Autodesk Inventor part; units mm, degrees
(part 2 of 2)
sketch "Sketch2" plane through (0, 0, 2.286) normal (0, 0, 1) x (1, 0, 0)
  line L0 (711.2, 0) -> (711.2, -863.6) projected
  line L1 (0, 0) -> (711.2, 0) projected
  line L2 (0, -863.6) -> (0, 0) projected
  point P0 (12.7, -12.7)
  point P1 (114.3, -12.7)
  point P2 (596.9, -12.7)
  point P3 (698.5, -12.7)
  point P4 (12.7, -38.1)
  point P5 (114.3, -38.1)
  point P6 (596.9, -38.1)
  point P7 (698.5, -38.1)
  point P8 (12.7, -63.5)
  point P9 (114.3, -63.5)
  point P10 (596.9, -63.5)
  point P11 (698.5, -63.5)
  point P12 (12.7, -88.9)
  point P13 (114.3, -88.9)
  point P14 (596.9, -88.9)
  point P15 (698.5, -88.9)
  point P16 (12.7, -114.3)
  point P17 (114.3, -114.3)
  point P18 (596.9, -114.3)
  point P19 (698.5, -114.3)
  point P20 (12.7, -139.7)
  point P21 (114.3, -139.7)
  point P22 (596.9, -139.7)
  point P23 (698.5, -139.7)
  point P24 (12.7, -165.1)
  point P25 (114.3, -165.1)
  point P26 (596.9, -165.1)
  point P27 (698.5, -165.1)
  point P28 (12.7, -190.5)
  point P29 (114.3, -190.5)
  point P30 (596.9, -190.5)
  point P31 (698.5, -190.5)
  point P32 (12.7, -215.9)
  point P33 (114.3, -215.9)
  point P34 (596.9, -215.9)
  point P35 (698.5, -215.9)
  point P36 (12.7, -241.3)
  point P37 (114.3, -241.3)
  point P38 (596.9, -241.3)
  point P39 (698.5, -241.3)
  point P40 (12.7, -266.7)
  point P41 (114.3, -266.7)
  point P42 (596.9, -266.7)
  point P43 (698.5, -266.7)
  point P44 (12.7, -292.1)
  point P45 (114.3, -292.1)
  point P46 (596.9, -292.1)
  point P47 (698.5, -292.1)
  point P48 (12.7, -317.5)
  point P49 (114.3, -317.5)
  point P50 (596.9, -317.5)
  point P51 (698.5, -317.5)
  point P52 (12.7, -342.9)
  point P53 (114.3, -342.9)
  point P54 (596.9, -342.9)
  point P55 (698.5, -342.9)
  point P56 (12.7, -368.3)
  point P57 (114.3, -368.3)
  point P58 (596.9, -368.3)
  point P59 (698.5, -368.3)
  point P60 (12.7, -393.7)
  point P61 (114.3, -393.7)
  point P62 (596.9, -393.7)
  point P63 (698.5, -393.7)
  point P64 (12.7, -419.1)
  point P65 (114.3, -419.1)
  point P66 (596.9, -419.1)
  point P67 (698.5, -419.1)
  point P68 (12.7, -444.5)
  point P69 (114.3, -444.5)
  point P70 (596.9, -444.5)
  point P71 (698.5, -444.5)
  point P72 (12.7, -469.9)
  point P73 (114.3, -469.9)
  point P74 (596.9, -469.9)
  point P75 (698.5, -469.9)
  point P76 (12.7, -495.3)
  point P77 (114.3, -495.3)
  point P78 (596.9, -495.3)
  point P79 (698.5, -495.3)
  point P80 (12.7, -520.7)
  point P81 (114.3, -520.7)
  point P82 (596.9, -520.7)
  point P83 (698.5, -520.7)
  point P84 (12.7, -546.1)
  point P85 (114.3, -546.1)
  point P86 (596.9, -546.1)
  point P87 (698.5, -546.1)
  point P88 (12.7, -571.5)
  point P89 (114.3, -571.5)
  point P90 (596.9, -571.5)
  point P91 (698.5, -571.5)
  point P92 (12.7, -596.9)
  point P93 (114.3, -596.9)
  point P94 (596.9, -596.9)
  point P95 (698.5, -596.9)
  point P96 (12.7, -622.3)
  point P97 (114.3, -622.3)
  point P98 (596.9, -622.3)
  point P99 (698.5, -622.3)
  point P100 (12.7, -647.7)
  point P101 (114.3, -647.7)
  point P102 (596.9, -647.7)
  point P103 (698.5, -647.7)
  point P104 (12.7, -673.1)
  point P105 (114.3, -673.1)
  point P106 (596.9, -673.1)
  point P107 (698.5, -673.1)
  point P108 (12.7, -698.5)
  point P109 (114.3, -698.5)
  point P110 (596.9, -698.5)
  point P111 (698.5, -698.5)
  point P112 (12.7, -723.9)
  point P113 (114.3, -723.9)
  point P114 (596.9, -723.9)
  point P115 (698.5, -723.9)
  point P116 (12.7, -749.3)
  point P117 (114.3, -749.3)
  point P118 (596.9, -749.3)
  point P119 (698.5, -749.3)
  point P120 (12.7, -774.7)
  point P121 (114.3, -774.7)
  point P122 (596.9, -774.7)
  point P123 (698.5, -774.7)
  point P124 (12.7, -800.1)
  point P125 (114.3, -800.1)
  point P126 (596.9, -800.1)
  point P127 (698.5, -800.1)
  point P128 (12.7, -825.5)
  point P129 (114.3, -825.5)
  point P130 (596.9, -825.5)
  point P131 (698.5, -825.5)
  point P132 (12.7, -850.9)
  point P133 (114.3, -850.9)
  point P134 (596.9, -850.9)
  point P135 (698.5, -850.9)
  dimension "d37" = 12.7
  dimension "d38" = 114.3
  dimension "d39" = 114.3
  dimension "d40" = 12.7
  dimension "d41" = 12.7
  dimension "d44" = 25.4
  constraints: 3 horizontal alignment, 1 vertical, 132 other
  measures "d37" distance from line of L2 point (12.7, -12.7)
  measures "d38" distance from line of L2 point (114.3, -12.7)
  measures "d39" distance from line of L0 point (596.9, -12.7)
  measures "d40" distance from line of L0 point (698.5, -12.7)
  measures "d41" distance from line of L1 point (698.5, -12.7)
  measures "d44" distance of point (698.5, -12.7) point (698.5, -38.1)
hole "Hole1" at (12.7, -12.7, 2.286) at (114.3, -12.7, 2.286) at (596.9, -12.7, 2.286) at (698.5, -12.7, 2.286) at (698.5, -38.1, 2.286) at (596.9, -38.1, 2.286) at (114.3, -38.1, 2.286) at (12.7, -38.1, 2.286) at (698.5, -63.5, 2.286) at (596.9, -63.5, 2.286) at (114.3, -63.5, 2.286) at (12.7, -63.5, 2.286) at (698.5, -88.9, 2.286) at (596.9, -88.9, 2.286) at (114.3, -88.9, 2.286) at (12.7, -88.9, 2.286) at (698.5, -114.3, 2.286) at (596.9, -114.3, 2.286) at (114.3, -114.3, 2.286) at (12.7, -114.3, 2.286) at (698.5, -139.7, 2.286) at (596.9, -139.7, 2.286) at (114.3, -139.7, 2.286) at (12.7, -139.7, 2.286) at (698.5, -165.1, 2.286) at (596.9, -165.1, 2.286) at (114.3, -165.1, 2.286) at (12.7, -165.1, 2.286) at (698.5, -190.5, 2.286) at (596.9, -190.5, 2.286) at (114.3, -190.5, 2.286) at (12.7, -190.5, 2.286) at (698.5, -215.9, 2.286) at (596.9, -215.9, 2.286) at (114.3, -215.9, 2.286) at (12.7, -215.9, 2.286) at (698.5, -241.3, 2.286) at (596.9, -241.3, 2.286) at (114.3, -241.3, 2.286) at (12.7, -241.3, 2.286) at (698.5, -266.7, 2.286) at (596.9, -266.7, 2.286) at (114.3, -266.7, 2.286) at (12.7, -266.7, 2.286) at (698.5, -292.1, 2.286) at (596.9, -292.1, 2.286) at (114.3, -292.1, 2.286) at (12.7, -292.1, 2.286) at (698.5, -317.5, 2.286) at (596.9, -317.5, 2.286) direction (0, 0, -1) diameter 6.7564 end through all and at (114.3, -317.5, 2.286) (12.7, -317.5, 2.286) (698.5, -342.9, 2.286) (596.9, -342.9, 2.286) (114.3, -342.9, 2.286) (12.7, -342.9, 2.286) (698.5, -368.3, 2.286) (596.9, -368.3, 2.286) (114.3, -368.3, 2.286) (12.7, -368.3, 2.286) (698.5, -393.7, 2.286) (596.9, -393.7, 2.286) (114.3, -393.7, 2.286) (12.7, -393.7, 2.286) (698.5, -419.1, 2.286) (596.9, -419.1, 2.286) (114.3, -419.1, 2.286) (12.7, -419.1, 2.286) (698.5, -444.5, 2.286) (596.9, -444.5, 2.286) (114.3, -444.5, 2.286) (12.7, -444.5, 2.286) (698.5, -469.9, 2.286) (596.9, -469.9, 2.286) (114.3, -469.9, 2.286) (12.7, -469.9, 2.286) (698.5, -495.3, 2.286) (596.9, -495.3, 2.286) (114.3, -495.3, 2.286) (12.7, -495.3, 2.286) (698.5, -520.7, 2.286) (596.9, -520.7, 2.286) (114.3, -520.7, 2.286) (12.7, -520.7, 2.286) (698.5, -546.1, 2.286) (596.9, -546.1, 2.286) (114.3, -546.1, 2.286) (12.7, -546.1, 2.286) (698.5, -571.5, 2.286) (596.9, -571.5, 2.286) (114.3, -571.5, 2.286) (12.7, -571.5, 2.286) (698.5, -596.9, 2.286) (596.9, -596.9, 2.286) (114.3, -596.9, 2.286) (12.7, -596.9, 2.286) (698.5, -622.3, 2.286) (596.9, -622.3, 2.286) (114.3, -622.3, 2.286) (12.7, -622.3, 2.286) (698.5, -647.7, 2.286) (596.9, -647.7, 2.286) (114.3, -647.7, 2.286) (12.7, -647.7, 2.286) (698.5, -673.1, 2.286) (596.9, -673.1, 2.286) (114.3, -673.1, 2.286) (12.7, -673.1, 2.286) (698.5, -698.5, 2.286) (596.9, -698.5, 2.286) (114.3, -698.5, 2.286) (12.7, -698.5, 2.286) (698.5, -723.9, 2.286) (596.9, -723.9, 2.286) (114.3, -723.9, 2.286) (12.7, -723.9, 2.286) (698.5, -749.3, 2.286) (596.9, -749.3, 2.286) (114.3, -749.3, 2.286) (12.7, -749.3, 2.286) (698.5, -774.7, 2.286) (596.9, -774.7, 2.286) (114.3, -774.7, 2.286) (12.7, -774.7, 2.286) (698.5, -800.1, 2.286) (596.9, -800.1, 2.286) (114.3, -800.1, 2.286) (12.7, -800.1, 2.286) (698.5, -825.5, 2.286) (596.9, -825.5, 2.286) (114.3, -825.5, 2.286) (12.7, -825.5, 2.286) (698.5, -850.9, 2.286) (596.9, -850.9, 2.286) (114.3, -850.9, 2.286) (12.7, -850.9, 2.286)
sketch "Sketch3" plane through (0, 0, 2.286) normal (0, 0, 1) x (1, 0, 0)
  line L0 (0, 0) -> (711.2, 0) projected
  line L1 (0, -863.6) -> (0, 0) projected
  line L2 (34.925, -38.1) -> (92.075, -38.1)
  line L3 (95.25, -41.275) -> (95.25, -161.925)
  line L4 (92.075, -165.1) -> (34.925, -165.1)
  line L5 (31.75, -161.925) -> (31.75, -41.275)
  arc A0 (34.925, -38.1) -> (31.75, -41.275) centre (34.925, -41.275) ccw
  arc A1 (31.75, -161.925) -> (34.925, -165.1) centre (34.925, -161.925) ccw
  arc A2 (92.075, -165.1) -> (95.25, -161.925) centre (92.075, -161.925) ccw
  arc A3 (95.25, -41.275) -> (92.075, -38.1) centre (92.075, -41.275) ccw
  line L6 (34.925, -203.2) -> (92.075, -203.2)
  line L7 (95.25, -206.375) -> (95.25, -327.025)
  line L8 (92.075, -330.2) -> (34.925, -330.2)
  line L9 (31.75, -327.025) -> (31.75, -206.375)
  arc A4 (34.925, -203.2) -> (31.75, -206.375) centre (34.925, -206.375) ccw
  arc A5 (31.75, -327.025) -> (34.925, -330.2) centre (34.925, -327.025) ccw
  arc A6 (92.075, -330.2) -> (95.25, -327.025) centre (92.075, -327.025) ccw
  arc A7 (95.25, -206.375) -> (92.075, -203.2) centre (92.075, -206.375) ccw
  line L10 (34.925, -368.3) -> (92.075, -368.3)
  line L11 (95.25, -371.475) -> (95.25, -492.125)
  line L12 (92.075, -495.3) -> (34.925, -495.3)
  line L13 (31.75, -492.125) -> (31.75, -371.475)
  arc A8 (34.925, -368.3) -> (31.75, -371.475) centre (34.925, -371.475) ccw
  arc A9 (31.75, -492.125) -> (34.925, -495.3) centre (34.925, -492.125) ccw
  arc A10 (92.075, -495.3) -> (95.25, -492.125) centre (92.075, -492.125) ccw
  arc A11 (95.25, -371.475) -> (92.075, -368.3) centre (92.075, -371.475) ccw
  line L14 (34.925, -533.4) -> (92.075, -533.4)
  line L15 (95.25, -536.575) -> (95.25, -657.225)
  line L16 (92.075, -660.4) -> (34.925, -660.4)
  line L17 (31.75, -657.225) -> (31.75, -536.575)
  arc A12 (34.925, -533.4) -> (31.75, -536.575) centre (34.925, -536.575) ccw
  arc A13 (31.75, -657.225) -> (34.925, -660.4) centre (34.925, -657.225) ccw
  arc A14 (92.075, -660.4) -> (95.25, -657.225) centre (92.075, -657.225) ccw
  arc A15 (95.25, -536.575) -> (92.075, -533.4) centre (92.075, -536.575) ccw
  line L18 (34.925, -698.5) -> (92.075, -698.5)
  line L19 (95.25, -701.675) -> (95.25, -822.325)
  line L20 (92.075, -825.5) -> (34.925, -825.5)
  line L21 (31.75, -822.325) -> (31.75, -701.675)
  arc A16 (34.925, -698.5) -> (31.75, -701.675) centre (34.925, -701.675) ccw
  arc A17 (31.75, -822.325) -> (34.925, -825.5) centre (34.925, -822.325) ccw
  arc A18 (92.075, -825.5) -> (95.25, -822.325) centre (92.075, -822.325) ccw
  arc A19 (95.25, -701.675) -> (92.075, -698.5) centre (92.075, -701.675) ccw
  line L22 (619.125, -38.1) -> (676.275, -38.1)
  line L23 (679.45, -41.275) -> (679.45, -161.925)
  line L24 (676.275, -165.1) -> (619.125, -165.1)
  line L25 (615.95, -161.925) -> (615.95, -41.275)
  arc A20 (619.125, -38.1) -> (615.95, -41.275) centre (619.125, -41.275) ccw
  arc A21 (615.95, -161.925) -> (619.125, -165.1) centre (619.125, -161.925) ccw
  arc A22 (676.275, -165.1) -> (679.45, -161.925) centre (676.275, -161.925) ccw
  arc A23 (679.45, -41.275) -> (676.275, -38.1) centre (676.275, -41.275) ccw
  line L26 (619.125, -203.2) -> (676.275, -203.2)
  line L27 (679.45, -206.375) -> (679.45, -327.025)
  line L28 (676.275, -330.2) -> (619.125, -330.2)
  line L29 (615.95, -327.025) -> (615.95, -206.375)
  arc A24 (619.125, -203.2) -> (615.95, -206.375) centre (619.125, -206.375) ccw
  arc A25 (615.95, -327.025) -> (619.125, -330.2) centre (619.125, -327.025) ccw
  arc A26 (676.275, -330.2) -> (679.45, -327.025) centre (676.275, -327.025) ccw
  arc A27 (679.45, -206.375) -> (676.275, -203.2) centre (676.275, -206.375) ccw
  line L30 (619.125, -368.3) -> (676.275, -368.3)
  line L31 (679.45, -371.475) -> (679.45, -492.125)
  line L32 (676.275, -495.3) -> (619.125, -495.3)
  line L33 (615.95, -492.125) -> (615.95, -371.475)
  arc A28 (619.125, -368.3) -> (615.95, -371.475) centre (619.125, -371.475) ccw
  arc A29 (615.95, -492.125) -> (619.125, -495.3) centre (619.125, -492.125) ccw
  arc A30 (676.275, -495.3) -> (679.45, -492.125) centre (676.275, -492.125) ccw
  arc A31 (679.45, -371.475) -> (676.275, -368.3) centre (676.275, -371.475) ccw
  line L34 (619.125, -533.4) -> (676.275, -533.4)
  line L35 (679.45, -536.575) -> (679.45, -657.225)
  line L36 (676.275, -660.4) -> (619.125, -660.4)
  line L37 (615.95, -657.225) -> (615.95, -536.575)
  arc A32 (619.125, -533.4) -> (615.95, -536.575) centre (619.125, -536.575) ccw
  arc A33 (615.95, -657.225) -> (619.125, -660.4) centre (619.125, -657.225) ccw
  arc A34 (676.275, -660.4) -> (679.45, -657.225) centre (676.275, -657.225) ccw
  arc A35 (679.45, -536.575) -> (676.275, -533.4) centre (676.275, -536.575) ccw
  line L38 (619.125, -698.5) -> (676.275, -698.5)
  line L39 (679.45, -701.675) -> (679.45, -822.325)
  line L40 (676.275, -825.5) -> (619.125, -825.5)
  line L41 (615.95, -822.325) -> (615.95, -701.675)
  arc A36 (619.125, -698.5) -> (615.95, -701.675) centre (619.125, -701.675) ccw
  arc A37 (615.95, -822.325) -> (619.125, -825.5) centre (619.125, -822.325) ccw
  arc A38 (676.275, -825.5) -> (679.45, -822.325) centre (676.275, -822.325) ccw
  arc A39 (679.45, -701.675) -> (676.275, -698.5) centre (676.275, -701.675) ccw
  point P0 (31.75, -38.1)
  point P1 (31.75, -165.1)
  point P2 (31.75, -203.2)
  point P3 (31.75, -330.2)
  point P4 (31.75, -368.3)
  point P5 (31.75, -495.3)
  point P6 (31.75, -533.4)
  point P7 (31.75, -660.4)
  point P8 (31.75, -698.5)
  point P9 (31.75, -825.5)
  point P10 (615.95, -38.1)
  point P11 (615.95, -165.1)
  point P12 (615.95, -203.2)
  point P13 (615.95, -330.2)
  point P14 (615.95, -368.3)
  point P15 (615.95, -495.3)
  point P16 (615.95, -533.4)
  point P17 (615.95, -660.4)
  point P18 (615.95, -698.5)
  point P19 (615.95, -825.5)
  dimension "d56" = 31.75
  dimension "d57" = 38.1
  dimension "d58" = 95.25
  dimension "d59" = 127
  dimension "d60" = 3.175
  dimension "d63" = 165.1
  dimension "d66" = 584.2
  constraints: 80 end point, 80 point on circle, 40 centre point, 40 point on line, 8 tangent, 3 equal radius, 2 horizontal, 2 parallel, 1 perpendicular, 1 vertical, 198 other
  measures "d56" distance between parallel lines of L1 L5
  measures "d57" distance between parallel lines of L0 L2
  measures "d58" distance between parallel lines of L1 L3
  measures "d59" distance of point (31.75, -165.1) point (31.75, -38.1)
  measures "d60" radius of A0
  measures "d63" distance of point (31.75, -165.1) point (31.75, -330.2)
  measures "d66" distance of point (31.75, -165.1) point (615.95, -165.1)
extrude "Cut1" cut sketch "Sketch3" against normal blind 3.048
sketch "Sketch4" plane through (0, 0, 2.286) normal (0, 0, 1) x (1, 0, 0)
  line L0 (190.5, -234.8865) -> (142.9908, -163.6227) projected
  arc A0 (145.6325, -158.6865) -> (142.9908, -163.6227) centre (145.6325, -161.8615) ccw projected
  line L1 (145.6325, -158.6865) -> (187.325, -158.6865) projected
  arc A1 (190.5, -161.8615) -> (187.325, -158.6865) centre (187.325, -161.8615) ccw projected
  line L2 (190.5, -161.8615) -> (190.5, -234.8865) projected
  arc A2 (187.325, -145.9865) -> (190.5, -142.8115) centre (187.325, -142.8115) ccw projected
  line L3 (187.325, -145.9865) -> (145.6325, -145.9865) projected
  arc A3 (142.9908, -141.0503) -> (145.6325, -145.9865) centre (145.6325, -142.8115) ccw projected
  line L4 (142.9908, -141.0503) -> (190.5, -69.7865) projected
  line L5 (190.5, -69.7865) -> (190.5, -142.8115) projected
  arc A4 (571.5, -161.8615) -> (568.325, -158.6865) centre (568.325, -161.8615) ccw projected
  line L6 (571.5, -161.8615) -> (571.5, -224.4002) projected
  arc A5 (565.6832, -226.1614) -> (571.5, -224.4002) centre (568.325, -224.4002) ccw projected
  line L7 (565.6832, -226.1614) -> (523.9908, -163.6227) projected
  arc A6 (526.6325, -158.6865) -> (523.9908, -163.6227) centre (526.6325, -161.8615) ccw projected
  line L8 (526.6325, -158.6865) -> (568.325, -158.6865) projected
  arc A7 (142.875, -46.9011) -> (139.7, -50.0761) centre (142.875, -50.0761) ccw projected
  line L9 (142.875, -46.9011) -> (184.5675, -46.9011) projected
  arc A8 (187.2092, -51.8373) -> (184.5675, -46.9011) centre (184.5675, -50.0761) ccw projected
  line L10 (187.2092, -51.8373) -> (145.5168, -114.376) projected
  arc A9 (139.7, -112.6148) -> (145.5168, -114.376) centre (142.875, -112.6148) ccw projected
  line L11 (139.7, -112.6148) -> (139.7, -50.0761) projected
  arc A10 (523.875, -46.9011) -> (520.7, -50.0761) centre (523.875, -50.0761) ccw projected
  line L12 (523.875, -46.9011) -> (565.5675, -46.9011) projected
  arc A11 (568.2092, -51.8373) -> (565.5675, -46.9011) centre (565.5675, -50.0761) ccw projected
  line L13 (568.2092, -51.8373) -> (526.5168, -114.376) projected
  arc A12 (520.7, -112.6148) -> (526.5168, -114.376) centre (523.875, -112.6148) ccw projected
  line L14 (520.7, -112.6148) -> (520.7, -50.0761) projected
  arc A13 (568.325, -145.9865) -> (571.5, -142.8115) centre (568.325, -142.8115) ccw projected
  line L15 (568.325, -145.9865) -> (526.6325, -145.9865) projected
  arc A14 (523.9908, -141.0503) -> (526.6325, -145.9865) centre (526.6325, -142.8115) ccw projected
  line L16 (523.9908, -141.0503) -> (565.6832, -78.5116) projected
  arc A15 (571.5, -80.2728) -> (565.6832, -78.5116) centre (568.325, -80.2728) ccw projected
  line L17 (571.5, -80.2728) -> (571.5, -142.8115) projected
  arc A16 (565.5675, -257.7719) -> (568.2092, -252.8357) centre (565.5675, -254.5969) ccw projected
  line L18 (565.5675, -257.7719) -> (523.875, -257.7719) projected
  arc A17 (520.7, -254.5969) -> (523.875, -257.7719) centre (523.875, -254.5969) ccw projected
  line L19 (520.7, -254.5969) -> (520.7, -192.0582) projected
  arc A18 (526.5168, -190.297) -> (520.7, -192.0582) centre (523.875, -192.0582) ccw projected
  line L20 (526.5168, -190.297) -> (568.2092, -252.8357) projected
  arc A19 (184.5675, -257.7719) -> (187.2092, -252.8357) centre (184.5675, -254.5969) ccw projected
  line L21 (184.5675, -257.7719) -> (142.875, -257.7719) projected
  arc A20 (139.7, -254.5969) -> (142.875, -257.7719) centre (142.875, -254.5969) ccw projected
  line L22 (139.7, -254.5969) -> (139.7, -192.0582) projected
  arc A21 (145.5168, -190.297) -> (139.7, -192.0582) centre (142.875, -192.0582) ccw projected
  line L23 (145.5168, -190.297) -> (187.2092, -252.8357) projected
  line L24 (0, 0) -> (711.2, 0) projected
  line L25 (0, -863.6) -> (0, 0) projected
  line L26 (711.2, -863.6) -> (0, -863.6) projected
  line L27 (523.875, -46.9011) -> (568.325, -46.9011)
  line L28 (571.5, -50.0761) -> (571.5, -254.5969)
  line L29 (568.325, -257.7719) -> (523.875, -257.7719)
  line L30 (520.7, -254.5969) -> (520.7, -50.0761)
  arc A22 (523.875, -46.9011) -> (520.7, -50.0761) centre (523.875, -50.0761) ccw
  arc A23 (571.5, -50.0761) -> (568.325, -46.9011) centre (568.325, -50.0761) ccw
  arc A24 (520.7, -254.5969) -> (523.875, -257.7719) centre (523.875, -254.5969) ccw
  arc A25 (568.325, -257.7719) -> (571.5, -254.5969) centre (568.325, -254.5969) ccw
  line L31 (355.6, 0) -> (355.6, -863.6) construction
  line L32 (139.7, -50.0761) -> (139.7, -254.5969)
  line L33 (142.875, -257.7719) -> (187.325, -257.7719)
  line L34 (190.5, -254.5969) -> (190.5, -50.0761)
  line L35 (187.325, -46.9011) -> (142.875, -46.9011)
  arc A26 (142.875, -46.9011) -> (139.7, -50.0761) centre (142.875, -50.0761) ccw
  arc A27 (190.5, -50.0761) -> (187.325, -46.9011) centre (187.325, -50.0761) ccw
  arc A28 (139.7, -254.5969) -> (142.875, -257.7719) centre (142.875, -254.5969) ccw
  arc A29 (187.325, -257.7719) -> (190.5, -254.5969) centre (187.325, -254.5969) ccw
  point P0 (139.7, -257.7719)
  dimension "d71" = 0
  dimension "d72" = 0
  dimension "d73" = 0
  dimension "d74" = 0
  dimension "d75" = 3.175
  dimension "d76" = 355.6
  dimension "d77" = 0
  dimension "d78" = 0
  dimension "d79" = 0
  dimension "d80" = 3.175
  constraints: 18 end point, 16 point on circle, 16 tangent, 8 centre point, 6 equal radius, 3 point on line, 2 collinear, 2 midpoint, 2 parallel, 2 perpendicular, 1 horizontal, 1 vertical
  measures "d71" distance between parallel lines of L14 L30
  measures "d72" distance between parallel lines of L17 L28
  measures "d73" distance between parallel lines of L18 L29
  measures "d74" distance between parallel lines of L12 L27
  measures "d75" radius of A22
  measures "d76" distance between parallel lines of L25 L31
  measures "d77" distance between parallel lines of L5 L34
  measures "d78" distance between parallel lines of L9 L35
  measures "d79" distance between parallel lines of L33 L21
  measures "d80" radius of A26
extrude "Cut2" cut sketch "Sketch4" against normal blind 3.048 contours L34 A29 L33 A19 L23 A21 L32 A9 L10 A8 L35 A27 L4 A3 L3 A2 A1 L1 A0 L0 | A4 L8 A6 L7 A5 L28 A25 L29 A16 L20 A18 L30 A12 L13 A11 L27 A23 A15 L16 A14 L15 A13
sketch "Sketch5" plane through (0, 0, 2.286) normal (0, 0, 1) x (1, 0, 0)
  circle A0 centre (12.7, -850.9) radius 3.3782 projected
  circle A1 centre (114.3, -850.9) radius 3.3782 projected
  circle A2 centre (596.9, -850.9) radius 3.3782 projected
  circle A3 centre (698.5, -850.9) radius 3.3782 projected
  circle A4 centre (12.7, -825.5) radius 3.3782 projected
  circle A5 centre (114.3, -825.5) radius 3.3782 projected
  circle A6 centre (596.9, -825.5) radius 3.3782 projected
  circle A7 centre (698.5, -825.5) radius 3.3782 projected
  circle A8 centre (12.7, -800.1) radius 3.3782 projected
  circle A9 centre (114.3, -800.1) radius 3.3782 projected
  circle A10 centre (596.9, -800.1) radius 3.3782 projected
  circle A11 centre (698.5, -800.1) radius 3.3782 projected
  circle A12 centre (12.7, -774.7) radius 3.3782 projected
  circle A13 centre (114.3, -774.7) radius 3.3782 projected
  circle A14 centre (596.9, -774.7) radius 3.3782 projected
  circle A15 centre (698.5, -774.7) radius 3.3782 projected
  circle A16 centre (12.7, -749.3) radius 3.3782 projected
  circle A17 centre (114.3, -749.3) radius 3.3782 projected
  circle A18 centre (596.9, -749.3) radius 3.3782 projected
  circle A19 centre (698.5, -749.3) radius 3.3782 projected
  circle A20 centre (12.7, -723.9) radius 3.3782 projected
  circle A21 centre (114.3, -723.9) radius 3.3782 projected
  circle A22 centre (596.9, -723.9) radius 3.3782 projected
  circle A23 centre (698.5, -723.9) radius 3.3782 projected
  circle A24 centre (12.7, -698.5) radius 3.3782 projected
  circle A25 centre (114.3, -698.5) radius 3.3782 projected
  circle A26 centre (596.9, -698.5) radius 3.3782 projected
  circle A27 centre (698.5, -698.5) radius 3.3782 projected
  circle A28 centre (12.7, -673.1) radius 3.3782 projected
  circle A29 centre (114.3, -673.1) radius 3.3782 projected
  circle A30 centre (596.9, -673.1) radius 3.3782 projected
  circle A31 centre (698.5, -673.1) radius 3.3782 projected
  circle A32 centre (12.7, -647.7) radius 3.3782 projected
  circle A33 centre (114.3, -647.7) radius 3.3782 projected
  circle A34 centre (596.9, -647.7) radius 3.3782 projected
  circle A35 centre (698.5, -647.7) radius 3.3782 projected
  circle A36 centre (12.7, -622.3) radius 3.3782 projected
  circle A37 centre (114.3, -622.3) radius 3.3782 projected
  circle A38 centre (596.9, -622.3) radius 3.3782 projected
  circle A39 centre (698.5, -622.3) radius 3.3782 projected
  circle A40 centre (12.7, -596.9) radius 3.3782 projected
  circle A41 centre (114.3, -596.9) radius 3.3782 projected
  circle A42 centre (596.9, -596.9) radius 3.3782 projected
  circle A43 centre (698.5, -596.9) radius 3.3782 projected
  circle A44 centre (12.7, -571.5) radius 3.3782 projected
  circle A45 centre (114.3, -571.5) radius 3.3782 projected
  circle A46 centre (596.9, -571.5) radius 3.3782 projected
  circle A47 centre (698.5, -571.5) radius 3.3782 projected
  circle A48 centre (12.7, -546.1) radius 3.3782 projected
  circle A49 centre (114.3, -546.1) radius 3.3782 projected
  circle A50 centre (596.9, -546.1) radius 3.3782 projected
  circle A51 centre (698.5, -546.1) radius 3.3782 projected
  circle A52 centre (12.7, -520.7) radius 3.3782 projected
  circle A53 centre (114.3, -520.7) radius 3.3782 projected
  circle A54 centre (596.9, -520.7) radius 3.3782 projected
  circle A55 centre (698.5, -520.7) radius 3.3782 projected
  circle A56 centre (12.7, -495.3) radius 3.3782 projected
  circle A57 centre (114.3, -495.3) radius 3.3782 projected
  circle A58 centre (596.9, -495.3) radius 3.3782 projected
  circle A59 centre (698.5, -495.3) radius 3.3782 projected
  circle A60 centre (12.7, -469.9) radius 3.3782 projected
  circle A61 centre (114.3, -469.9) radius 3.3782 projected
  circle A62 centre (596.9, -469.9) radius 3.3782 projected
  circle A63 centre (698.5, -469.9) radius 3.3782 projected
  circle A64 centre (12.7, -444.5) radius 3.3782 projected
  circle A65 centre (114.3, -444.5) radius 3.3782 projected
  circle A66 centre (596.9, -444.5) radius 3.3782 projected
  circle A67 centre (698.5, -444.5) radius 3.3782 projected
  circle A68 centre (12.7, -419.1) radius 3.3782 projected
  circle A69 centre (114.3, -419.1) radius 3.3782 projected
  circle A70 centre (596.9, -419.1) radius 3.3782 projected
  circle A71 centre (698.5, -419.1) radius 3.3782 projected
  circle A72 centre (12.7, -393.7) radius 3.3782 projected
  circle A73 centre (114.3, -393.7) radius 3.3782 projected
  circle A74 centre (596.9, -393.7) radius 3.3782 projected
  circle A75 centre (698.5, -393.7) radius 3.3782 projected
  circle A76 centre (12.7, -368.3) radius 3.3782 projected
  circle A77 centre (114.3, -368.3) radius 3.3782 projected
  circle A78 centre (596.9, -368.3) radius 3.3782 projected
  circle A79 centre (698.5, -368.3) radius 3.3782 projected
  circle A80 centre (12.7, -342.9) radius 3.3782 projected
  circle A81 centre (114.3, -342.9) radius 3.3782 projected
  circle A82 centre (596.9, -342.9) radius 3.3782 projected
  circle A83 centre (698.5, -342.9) radius 3.3782 projected
  circle A84 centre (12.7, -317.5) radius 3.3782 projected
  circle A85 centre (114.3, -317.5) radius 3.3782 projected
  circle A86 centre (596.9, -317.5) radius 3.3782 projected
  circle A87 centre (698.5, -317.5) radius 3.3782 projected
  circle A88 centre (12.7, -292.1) radius 3.3782 projected
  circle A89 centre (114.3, -292.1) radius 3.3782 projected
  circle A90 centre (596.9, -292.1) radius 3.3782 projected
  circle A91 centre (698.5, -292.1) radius 3.3782 projected
  circle A92 centre (12.7, -266.7) radius 3.3782 projected
  circle A93 centre (114.3, -266.7) radius 3.3782 projected
  circle A94 centre (596.9, -266.7) radius 3.3782 projected
  circle A95 centre (698.5, -266.7) radius 3.3782 projected
  circle A96 centre (12.7, -241.3) radius 3.3782 projected
  circle A97 centre (114.3, -241.3) radius 3.3782 projected
  circle A98 centre (596.9, -241.3) radius 3.3782 projected
  circle A99 centre (698.5, -241.3) radius 3.3782 projected
  circle A100 centre (12.7, -215.9) radius 3.3782 projected
  circle A101 centre (114.3, -215.9) radius 3.3782 projected
  circle A102 centre (596.9, -215.9) radius 3.3782 projected
  circle A103 centre (698.5, -215.9) radius 3.3782 projected
  circle A104 centre (12.7, -190.5) radius 3.3782 projected
  circle A105 centre (114.3, -190.5) radius 3.3782 projected
  circle A106 centre (596.9, -190.5) radius 3.3782 projected
  circle A107 centre (698.5, -190.5) radius 3.3782 projected
  circle A108 centre (12.7, -165.1) radius 3.3782 projected
  circle A109 centre (114.3, -165.1) radius 3.3782 projected
  circle A110 centre (596.9, -165.1) radius 3.3782 projected
  circle A111 centre (698.5, -165.1) radius 3.3782 projected
  circle A112 centre (12.7, -139.7) radius 3.3782 projected
  circle A113 centre (114.3, -139.7) radius 3.3782 projected
  circle A114 centre (596.9, -139.7) radius 3.3782 projected
  circle A115 centre (698.5, -139.7) radius 3.3782 projected
  circle A116 centre (12.7, -114.3) radius 3.3782 projected
  circle A117 centre (114.3, -114.3) radius 3.3782 projected
  circle A118 centre (596.9, -114.3) radius 3.3782 projected
  circle A119 centre (698.5, -114.3) radius 3.3782 projected
  circle A120 centre (12.7, -88.9) radius 3.3782 projected
  circle A121 centre (114.3, -88.9) radius 3.3782 projected
  circle A122 centre (596.9, -88.9) radius 3.3782 projected
  circle A123 centre (698.5, -88.9) radius 3.3782 projected
  circle A124 centre (12.7, -63.5) radius 3.3782 projected
  circle A125 centre (114.3, -63.5) radius 3.3782 projected
  circle A126 centre (596.9, -63.5) radius 3.3782 projected
  circle A127 centre (698.5, -63.5) radius 3.3782 projected
  circle A128 centre (12.7, -38.1) radius 3.3782 projected
  circle A129 centre (114.3, -38.1) radius 3.3782 projected
  circle A130 centre (596.9, -38.1) radius 3.3782 projected
  circle A131 centre (698.5, -38.1) radius 3.3782 projected
  circle A132 centre (698.5, -12.7) radius 3.3782 projected
  circle A133 centre (596.9, -12.7) radius 3.3782 projected
  circle A134 centre (114.3, -12.7) radius 3.3782 projected
  circle A135 centre (12.7, -12.7) radius 3.3782 projected
  line L0 (711.2, 0) -> (711.2, -863.6) projected
  line L1 (0, 0) -> (711.2, 0) projected
  line L2 (0, -863.6) -> (0, 0) projected
  line L3 (711.2, -863.6) -> (0, -863.6) projected
equation "\"BendRadius\" = Thickness"
equation "\"BendReliefWidth\" = Thickness"
equation "\"BendReliefDepth\" = 0.5 * Thickness"
equation "\"CornerReliefSize\" = 4 * Thickness"
equation "\"MinimumRemnant\" = 2 * Thickness"
equation "\"TransitionRadius\" = BendRadius"
equation "\"JacobiRadiusSize\" = BendRadius"
equation "\"GapSize\" = Thickness"
equation "\"d4\" = d2"
equation "\"d5\" = d3"
equation "\"Thickness\" = 3.048"
body "Solid1"
